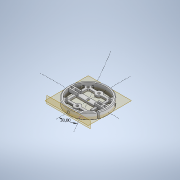
# Autodesk Inventor part: Electro_esp32_up
Saved by Autodesk Inventor 2020 (Build 240168000, 168)
## iProperties
Created: 2020-09-03
Part Number: Electro_esp32_up
Material: Generisch
Document SubType Name: Modeling
Designer: sp
Density: 1 g/cm^3
Appearance: Vorgabe
Author: sp
## iProperties of the stored document _3D-Druck.ipt
Created: 2020-09-03
Part Number: _3D-Druck
Material: Generisch
Document SubType Name: Modeling
Designer: sp
Density: 1 g/cm^3
Appearance: Vorgabe
Author: sp
Autodesk Inventor part; units mm, degrees
ref_plane "YZ Plane" through (0, 0, 0) normal (1, 0, 0) x (0, 1, 0)
sketch "Skizze1" plane through (0, 0, 0) normal (0, 1, 0) x (-1, 0, 0)
  circle A0 centre (0, 0) radius 30
  circle A1 centre (0, 0) radius 27
  dimension "d0" = 60
  dimension "d1" = 54
  constraints: 2 centre point, 2 coincident
  measures "d0" diameter of A0
  measures "d1" diameter of A1
extrude "Extrusion1" add sketch "Skizze1" along normal mid plane 10
ref_plane "Arbeitsebene1" through (0, 0, 0) normal (0, 1, 0) x (-1, 0, 0)
chamfer "Fase1" distance 1 angle 45 2 edges at (30, 5, 0) (30, -5, 0)
sketch "Skizze2" plane through (0, 0, 0) normal (0, 1, 0) x (-1, 0, 0)
  line L0 (0, 42.2301) -> (0, -36.7007) construction
  line L1 (32.6355, 0) -> (-32.6355, 0) construction
  line L2 (16.5, 34.419) -> (16.5, -40.3324) construction
  line L3 (-16.5, 35.4304) -> (-16.5, -34.8157) construction
  line L4 (23.5881, 16.5) -> (-32.0387, 16.5) construction
  line L5 (23.5881, -16.5) -> (-39.8541, -16.5) construction
  circle A0 centre (16.5, -16.5) radius 1.75
  circle A1 centre (16.5, 16.5) radius 1.75
  circle A2 centre (-16.5, 16.5) radius 1.75
  circle A3 centre (-16.5, -16.5) radius 1.75
  circle A4 centre (-16.5, 16.5) radius 3.6749
  circle A5 centre (-16.5, -16.5) radius 3.7161
  circle A6 centre (16.5, -16.5) radius 3.7
  circle A7 centre (16.5, 16.5) radius 3.6747
  point P0 (0, 0)
  dimension "d8" = 33
  dimension "d9" = 33
  dimension "d10" = 3.5
  dimension "d11" = 3.5
  dimension "d12" = 3.5
  dimension "d13" = 3.5
  constraints: 12 end point, 9 point on line, 8 centre point, 4 coincident, 3 horizontal, 3 vertical, 1 midpoint, 2 other
  measures "d8" distance between parallel lines of L3 L2
  measures "d9" distance between parallel lines of L4 L5
  measures "d10" diameter of A0
  measures "d11" diameter of A1
  measures "d12" diameter of A2
  measures "d13" diameter of A3
extrude "Extrusion2" add sketch "Skizze2" along normal mid plane 3
fillet "Rundung1" radius 2 16 edges at (-18.7043, 0.75, -19.4718) (-19.4718, 0.75, -18.7043) (-18.7043, -0.75, -19.4718) (-19.4718, -0.75, -18.7043) (-19.289, 0.75, 18.8927) (-18.8927, 0.75, 19.289) (-19.289, -0.75, 18.8927) (-18.8927, -0.75, 19.289) (18.8904, 0.75, 19.2913) (19.2913, 0.75, 18.8904) (18.8904, -0.75, 19.2913) (19.2913, -0.75, 18.8904) (19.551, 0.75, -18.6215) (18.6215, 0.75, -19.551) (19.551, -0.75, -18.6215) (18.6215, -0.75, -19.551)
sketch "Skizze3" plane through (0, 0, 0) normal (0, 1, 0) x (-1, 0, 0)
  circle A0 centre (-16.5, -16.5) radius 1.75 projected
  line L0 (16.5712, -18.25) -> (-16.5, -18.25)
  line L1 (-16.5, -18.25) -> (-16.5, -14.75)
  line L2 (-16.5, -14.75) -> (16.5712, -14.75)
  line L3 (16.5712, -14.75) -> (16.5712, -18.25)
  circle A1 centre (-16.5, 16.5) radius 1.75 projected
  line L4 (-18.25, 16.5) -> (-14.75, 16.5)
  line L5 (-14.75, 16.5) -> (-14.75, -16.5)
  line L6 (-14.75, -16.5) -> (-18.25, -16.5)
  line L7 (-18.25, -16.5) -> (-18.25, 16.5)
  circle A2 centre (16.5, 16.5) radius 1.75 projected
  line L8 (16.5, 14.75) -> (-16.8045, 14.75)
  line L9 (-16.8045, 14.75) -> (-16.8045, 18.2233)
  line L10 (-16.8045, 18.2233) -> (16.5, 18.2233)
  line L11 (16.5, 18.2233) -> (16.5, 14.75)
  circle A3 centre (-16.5, -16.5) radius 1.75 projected
  circle A4 centre (16.5, -16.5) radius 1.75 projected
  line L12 (18.25, -16.5) -> (14.75, -16.5)
  line L13 (14.75, -16.5) -> (14.75, 16.5)
  line L14 (14.75, 16.5) -> (18.25, 16.5)
  line L15 (18.25, 16.5) -> (18.25, -16.5)
  point P0 (0, 0)
  point P1 (14.75, -14.75)
  point P2 (-14.75, -14.75)
  point P3 (16.5, -18.25)
  point P4 (14.75, 14.75)
  point P5 (16.1955, 18.2233)
  point P6 (-16.1955, 18.2233)
  point P7 (-14.75, 14.75)
  point P8 (16.5712, -14.7514)
  point P9 (-16.8045, 14.7767)
  constraints: 32 end point, 8 parallel, 7 point on circle, 4 horizontal, 4 perpendicular, 2 other
extrude "Extrusion3" add sketch "Skizze3" against normal mid plane 3 contours L5 L2 L13 A4 L0 A0 | A0 L7 A1 L9 L8 L5 L2 | L13 L8 A2 L15 A4 L2 | L5 A1 L10 A2 L13 L8
ref_plane "Arbeitsebene2" through (0, 0, 30) normal (0, 0, 1) x (1, 0, 0)
sketch "Skizze4" plane through (0, 0, 30) normal (0, 0, 1) x (1, 0, 0)
  circle A0 centre (0, 0) radius 1.75
  dimension "d20" = 3.5
  constraints: 1 centre point, 1 coincident
  measures "d20" diameter of A0
extrude "Extrusion4" cut sketch "Skizze4" against normal blind 5
sketch "Skizze6" plane through (0, 0, 0) normal (0, 1, 0) x (-1, 0, 0)
  line L0 (0, 50.1563) -> (0, -65.6092) construction
  line L1 (-47.8971, 0) -> (73.2619, 0) construction
  line L2 (-30.0527, 52.0529) -> (47.8935, -82.954) construction
  point P0 (0, 0)
  point P1 (-14.9945, 25.9712)
  dimension "d24" = 30
  constraints: 6 end point, 4 point on line, 1 horizontal, 1 vertical
  measures "d24" angle of L2 L0
pattern_circular "Runde Anordnung2" count 3 over 360 about axis through (0, -10, 0) along (0, 1, 0) of "Extrusion4"
sketch "Skizze7" plane through (0, 0, 0) normal (0, 1, 0) x (-1, 0, 0)
  line L0 (28, -3.5) -> (13, -3.5)
  line L1 (13, -3.5) -> (13, -1.5)
  line L2 (13, -1.5) -> (28, -1.5)
  line L3 (28, -1.5) -> (28, -3.5)
  line L4 (28, 3.5) -> (13, 3.5)
  line L5 (13, 3.5) -> (13, 1.5)
  line L6 (13, 1.5) -> (28, 1.5)
  line L7 (28, 1.5) -> (28, 3.5)
  line L8 (47.9348, 0) -> (-36.1073, 0) construction
  line L9 (0, 34.6258) -> (0, -35.7568) construction
  line L10 (21, 3.5) -> (23, 3.5)
  line L11 (23, 3.5) -> (23, -3.5)
  line L12 (23, -3.5) -> (21, -3.5)
  line L13 (21, -3.5) -> (21, 3.5)
  point P0 (0, 0)
  point P1 (21, 1.5)
  point P2 (21, -1.5)
  point P3 (23, -1.5)
  point P4 (23, 1.5)
  dimension "d31" = 2
  dimension "d32" = 3
  dimension "d33" = 2
  dimension "d34" = 15
  dimension "d35" = 13
  dimension "d40" = 2
  dimension "d41" = 21
  constraints: 28 end point, 6 point on line, 5 parallel, 4 horizontal, 3 perpendicular, 1 vertical, 1 other
  measures "d31" distance of L4.end L5.end
  measures "d32" distance between parallel lines of L6 L2
  measures "d33" distance of L0.end L1.end
  measures "d34" distance of L0.start L0.end
  measures "d35" distance from line of point (0, 0) L5
  measures "d40" distance between parallel lines of L11 L13
  measures "d41" distance between parallel lines of L9 L13
extrude "Extrusion5" add sketch "Skizze7" along normal blind 5
mirror "Spiegeln1" about plane through (0, 0, 0) normal (1, 0, 0) of "Extrusion5"
sketch "Skizze8" plane through (0, -1.5, 0) normal (0, -1, 0) x (1, 0, 0)
  line L0 (-14.75, -13.24) -> (-14.75, 13.2687) projected
  line L1 (14.75, -13.2218) -> (14.75, -3.5) projected
  line L2 (-14.75, 3.5) -> (14.75, 3.5)
  line L3 (14.75, 3.5) -> (14.75, -3.5)
  line L4 (14.75, -3.5) -> (-14.75, -3.5)
  line L5 (-14.75, -3.5) -> (-14.75, 3.5)
  line L6 (-14.75, 3.5) -> (-13, 3.5) projected
  point P0 (0, 0)
  constraints: 8 end point, 2 parallel, 2 point on line, 1 horizontal, 1 perpendicular
extrude "Extrusion6" add sketch "Skizze8" against normal blind 3
sketch "Skizze9" plane through (0, -1.5, 0) normal (0, -1, 0) x (1, 0, 0)
  circle A0 centre (0, 0) radius 1.75
  dimension "d42" = 3.5
  constraints: 1 centre point, 1 coincident
  measures "d42" diameter of A0
extrude "Extrusion7" cut sketch "Skizze9" against normal blind 10
sketch "Skizze10" plane through (0, -1.5, 0) normal (0, -1, 0) x (1, 0, 0)
  circle A0 centre (0, 16.5) radius 1.75
  circle A1 centre (0, 16.5) radius 5
  point P0 (0, 0)
  dimension "d45" = 3.5
  dimension "d46" = 10
  constraints: 2 centre point, 1 coincident
  measures "d45" diameter of A0
  measures "d46" diameter of A1
extrude "Extrusion8" add sketch "Skizze10" against normal blind 3
sketch "Skizze11" plane through (0, -1.5, 0) normal (0, -1, 0) x (1, 0, 0)
  arc A0 (4.6936, 18.2233) -> (-4.6936, 18.2233) centre (0, 16.5) ccw projected
  circle A1 centre (0, 16.5) radius 1.75
  point P0 (0, 0)
  dimension "d49" = 3.5
  constraints: 1 centre point, 1 coincident
  measures "d49" diameter of A1
extrude "Extrusion9" cut sketch "Skizze11" against normal blind 3
mirror "Spiegeln2" about plane through (0, 0, 0) normal (0, 0, 1) of "Extrusion8"
mirror "Spiegeln3" about plane through (0, 0, 0) normal (0, 0, 1) of "Extrusion9"
sketch "Skizze12" plane through (0, -5, 0) normal (0, -1, 0) x (1, 0, 0)
  line L0 (14.75, 3.5) -> (14.75, 13.2685) projected
  line L1 (14.75, 13.2685) -> (31.4011, 13.2685)
  line L2 (31.4011, 13.2685) -> (31.4011, 11.2685)
  line L3 (31.4011, 11.2685) -> (14.75, 11.2685)
  line L4 (14.75, 11.2685) -> (14.75, 13.2685)
  point P0 (0, 0)
  dimension "d52" = 2
  constraints: 8 end point, 2 parallel, 1 horizontal, 1 perpendicular
  measures "d52" distance of L1.end L2.end
extrude "Extrusion10" cut sketch "Skizze12" against normal blind 10
